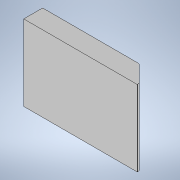
# Autodesk Inventor part: KabelBoxDeckel
Saved by Autodesk Inventor 2020.3 (Build 243373010, 373A)
## iProperties
Created: 2021-02-15
Part Number: KabelBoxDeckel
Material: Generisch
Document SubType Name: Modeling
Designer: Stefan
Density: 1 g/cm^3
Appearance: Vorgabe
Author: Stefan
Autodesk Inventor part; units mm, degrees
ref_plane "YZ Plane" through (0, 0, 0) normal (1, 0, 0) x (0, 1, 0)
ref_plane "XZ Plane" through (0, 0, 0) normal (0, 1, 0) x (-1, 0, 0)
ref_plane "XY Plane" through (0, 0, 0) normal (0, 0, 1) x (1, 0, 0)
sketch "Skizze1" plane through (0, 0, 0) normal (0, 0, 1) x (1, 0, 0)
  line L0 (-36.3412, 23.6948) -> (23.6588, 23.6948)
  line L1 (23.6588, 23.6948) -> (23.6588, -16.3052)
  line L2 (23.6588, -16.3052) -> (-36.3412, -16.3052)
  line L3 (-36.3412, -16.3052) -> (-36.3412, 23.6948)
  point P0 (0, 0)
  dimension "d0" = 60
  dimension "d1" = 40
  constraints: 8 end point, 2 parallel, 1 horizontal, 1 perpendicular
  measures "d0" distance of L1.end L2.end
  measures "d1" distance of L0.end L1.end
extrude "Extrusion1" add sketch "Skizze1" along normal blind 10
chamfer "Fase1" distance 9 angle 45 1 edges at (23.6588, 3.6948, 0)
fillet "Rundung1" radius 2 2 edges at (23.6588, 3.6948, 9) (14.6588, 3.6948, 0)
